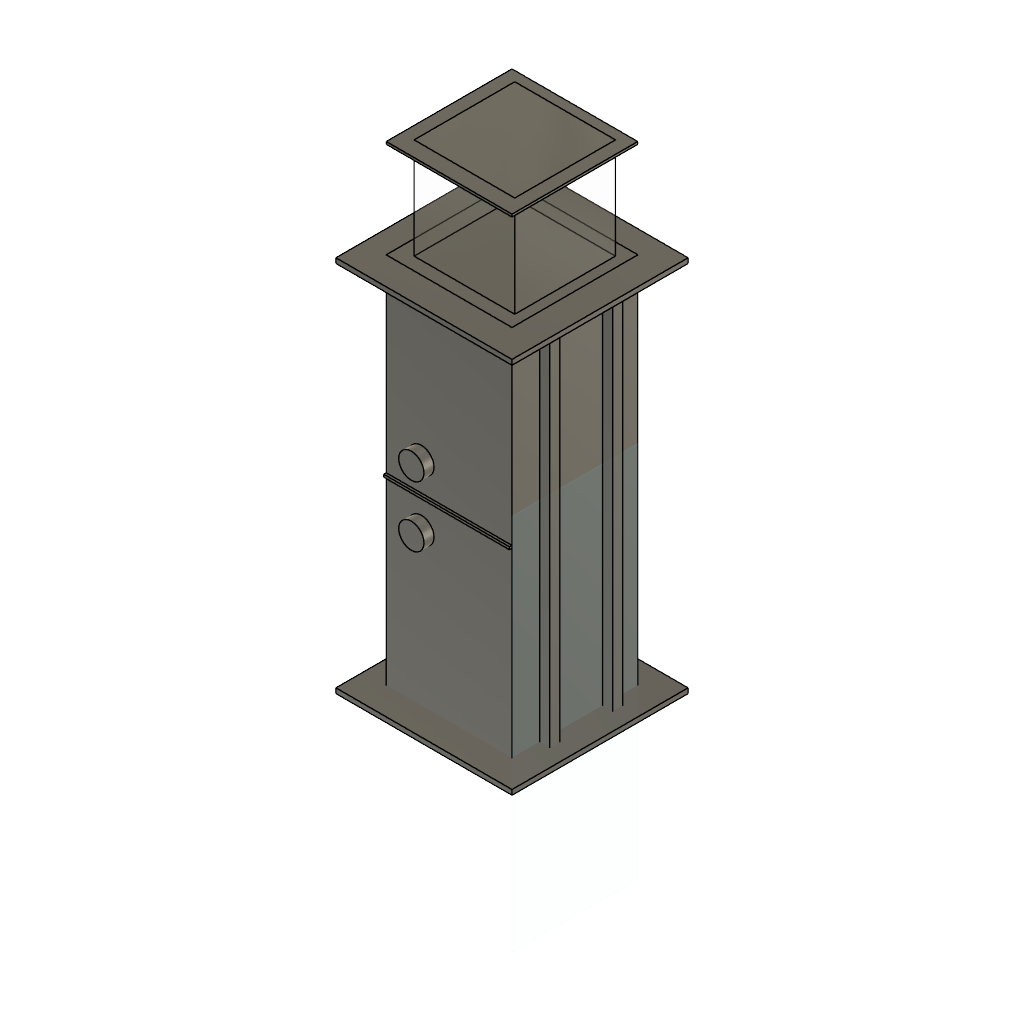
SolarPath+ (Autodesk Fusion 360 design; units mm, degrees)
Autodesk Fusion 360 part; units mm, degrees
sketch "Çizim1" plane through (0, 0, 0) normal (0, 1, 0) x (1, 0, 0)
  line L0 (0, 0) -> (250, 0)
  line L1 (250, 0) -> (250, 250)
  line L2 (250, 250) -> (0, 250)
  line L3 (0, 250) -> (0, 0)
  constraint horizontal L0
  constraint vertical L1
  constraint horizontal L2
  constraint vertical L3
  constraint coincident L0.start L3.end
extrude "Ekstrüzyon1" add sketch "Çizim1" along normal blind 750 makes body 1
move_body "Taşı1" bodies 1 to x (1, 0, 0) y (0, 1, 0) z (0, 0, 1) at (-125, 0, 250)
move_body "Taşı2" bodies 1 to x (1, 0, 0) y (0, 0, -1) z (0, 1, 0) at (0, 0, 0)
move_body "Taşı3" bodies 1 to x (1, 0, 0) y (0, 1, 0) z (0, 0, 1) at (0, -125, 750)
move_body "Taşı4" bodies 1 to x (1, 0, 0) y (0, 1, 0) z (0, 0, 1) at (0, 0, -325)
sketch "Çizim2" plane through (125, 0, 0) normal (1, 0, 0) x (0, 1, 0)
  line L0 (125, 425) -> (-125, 425)
  line L1 (-125, 425) -> (-125, -325)
  line L2 (-125, -325) -> (125, -325)
  line L3 (125, -325) -> (125, 425)
sketch "Çizim3" plane through (0, 0, 0) normal (0, 1, 0) x (1, 0, 0)
  line L0 (300, 150) -> (550, 150)
  line L1 (550, 150) -> (550, 155)
  line L2 (550, 155) -> (300, 155)
  line L3 (300, 155) -> (300, 150)
  constraint horizontal L0
  constraint vertical L1
  constraint horizontal L2
  constraint vertical L3
extrude "Ekstrüzyon2" add sketch "Çizim3" along normal blind 5 separate body makes body 2
sketch "Çizim4" plane through (0, 0, 0) normal (0, 1, 0) x (1, 0, 0)
move_body "Taşı5" bodies 2 to x (1, 0, 0) y (0, 1, 0) z (0, 0, 1) at (0, -135, 0)
move_body "Taşı6" bodies 2 to x (1, 0, 0) y (0, 1, 0) z (0, 0, 1) at (-425, 0, 0)
move_body "Taşı7" bodies 2 to x (1, 0, 0) y (0, 1, 0) z (0, 0, 1) at (0, 0, 150)
sketch "Çizim5" plane through (0, -125, 0) normal (0, -1, 0) x (1, 0, 0)
  line L0 (125, 425) -> (-125, 425)
  line L1 (-125, 425) -> (-125, -325)
  line L2 (-125, -325) -> (125, -325)
  line L3 (125, -325) -> (125, 425)
  line L4 (350, 0) -> (450, 0)
  line L5 (450, 0) -> (450, -35)
  line L6 (450, -35) -> (350, -35)
  line L7 (350, -35) -> (350, 0)
  dimension "d6" = 100
  dimension "d7" = 35
  constraint horizontal L4
  constraint vertical L5
  constraint horizontal L6
  constraint vertical L7
  measures "d6" distance of L4.start L4.end
  measures "d7" distance of L4.start L6.end
move_body "Taşı13" bodies 2 to x (1, 0, 0) y (0, 1, 0) z (0, 0, 1) at (0, 5, 70)
sketch "Çizim6" plane through (0, 0, 0) normal (0, 0, 1) x (1, 0, 0)
  line L0 (500, 150) -> (850, 150)
  line L1 (850, 150) -> (850, -200)
  line L2 (850, -200) -> (500, -200)
  line L3 (500, -200) -> (500, 150)
  constraint horizontal L0
  constraint vertical L1
  constraint horizontal L2
  constraint vertical L3
extrude "Ekstrüzyon4" add sketch "Çizim6" along normal blind 10 separate body makes body 3
move_body "Taşı16" bodies 3 to x (1, 0, 0) y (0, 1, 0) z (0, 0, 1) at (-670, 20, -330)
copy_body "Gövdeleri Kopyala Yapıştır2" bodies 3 makes body 4
move_body "Taşı17" bodies 4 to x (1, 0, 0) y (0, 1, 0) z (0, 0, 1) at (0, 0, 750)
sketch "Çizim7" plane through (0, 0, 0) normal (0, 1, 0) x (1, 0, 0)
  line L0 (450, 0) -> (650, 0)
  line L1 (650, 0) -> (650, -200)
  line L2 (650, -200) -> (450, -200)
  line L3 (450, -200) -> (450, 0)
  constraint horizontal L0
  constraint vertical L1
  constraint horizontal L2
  constraint vertical L3
extrude "Ekstrüzyon5" add sketch "Çizim7" along normal blind 200 separate body makes body 5
move_body "Taşı18" bodies 5 to x (1, 0, 0) y (0, 1, 0) z (0, 0, 1) at (-545, -99.5, 430)
sketch "Çizim8" plane through (0, 0, 0) normal (0, 1, 0) x (1, 0, 0)
  line L0 (500, 0) -> (750, 0)
  line L1 (750, 0) -> (750, -250)
  line L2 (750, -250) -> (500, -250)
  line L3 (500, -250) -> (500, 0)
  constraint horizontal L0
  constraint vertical L1
  constraint horizontal L2
  constraint vertical L3
extrude "Ekstrüzyon6" add sketch "Çizim8" along normal blind 5 separate body makes body 6
move_body "Taşı19" bodies 6 to x (1, 0, 0) y (0, 0, -1) z (0, 1, 0) at (0, -120, 130)
move_body "Taşı20" bodies 6 to x (1, 0, 0) y (0, 1, 0) z (0, 0, 1) at (-620, -10, 500)
move_body "Taşı21" bodies 3 to x (1, 0, 0) y (0, 1, 0) z (0, 0, 1) at (0, 0, 5)
move_body "Taşı22" bodies 4 to x (1, 0, 0) y (0, 1, 0) z (0, 0, 1) at (0, 0, -5)
move_body "Taşı23" bodies 5 to x (1, 0, 0) y (0, 1, 0) z (0, 0, 1) at (0, 0, -5)
move_body "Taşı24" bodies 6 to x (1, 0, 0) y (0, 1, 0) z (0, 0, 1) at (0, 0, -5)
sketch "Çizim9" plane through (0, 0, 0) normal (1, 0, 0) x (0, 1, 0)
sketch "Çizim10" plane through (0, 0, 0) normal (1, 0, 0) x (0, 1, 0)
  line L0 (500, 250) -> (520, 250)
  line L1 (520, 250) -> (520, -500)
  line L2 (520, -500) -> (500, -500)
  line L3 (500, -500) -> (500, 250)
  dimension "d16" = 20
  dimension "d17" = 750
  constraint horizontal L0
  constraint vertical L1
  constraint horizontal L2
  constraint vertical L3
  measures "d16" distance of L0.start L0.end
  measures "d17" distance of L0.start L2.end
sketch "Çizim11" plane through (0, 0, 0) normal (1, 0, 0) x (0, 1, 0)
  line L0 (-200, 420) -> (-220, 420)
  line L1 (-220, 420) -> (-220, -320)
  line L2 (-220, -320) -> (-200, -320)
  line L3 (-200, -320) -> (-200, 420)
  constraint horizontal L0
  constraint vertical L1
  constraint horizontal L2
  constraint vertical L3
extrude "Ekstrüzyon8" add sketch "Çizim11" along normal blind 20 separate body makes body 7
copy_body "Gövdeleri Kopyala Yapıştır7" bodies 7 makes body 8
move_body "Taşı32" bodies 8 to x (1, 0, 0) y (0, 1, 0) z (0, 0, 1) at (-200, 95, 0)
move_body "Taşı33" bodies 8 to x (1, 0, 0) y (0, 1, 0) z (0, 0, 1) at (0, 50, 0)
move_body "Taşı34" bodies 8 to x (1, 0, 0) y (0, 1, 0) z (0, 0, 1) at (55, 0, 0)
move_body "Taşı35" bodies 8 to x (1, 0, 0) y (0, 1, 0) z (0, 0, 1) at (5, 0, 0)
copy_body "Gövdeleri Kopyala Yapıştır8" bodies 7 makes body 9
move_body "Taşı36" bodies 9 to x (1, 0, 0) y (0, 1, 0) z (0, 0, 1) at (-145, 325, 0)
move_body "Taşı37" bodies 9 to x (1, 0, 0) y (0, 1, 0) z (0, 0, 1) at (0, -50, 0)
copy_body "Gövdeleri Kopyala Yapıştır9" bodies 7 makes body 10
move_body "Taşı38" bodies 10 to x (1, 0, 0) y (0, 1, 0) z (0, 0, 1) at (125, 100, 0)
move_body "Taşı39" bodies 10 to x (1, 0, 0) y (0, 1, 0) z (0, 0, 1) at (0, 50, 0)
copy_body "Gövdeleri Kopyala Yapıştır10" bodies 7 makes body 11
move_body "Taşı40" bodies 11 to x (1, 0, 0) y (0, 1, 0) z (0, 0, 1) at (200, 450, 0)
move_body "Taşı41" bodies 11 to x (1, 0, 0) y (0, 1, 0) z (0, 0, 1) at (-75, -125, 0)
move_body "Taşı42" bodies 11 to x (1, 0, 0) y (0, 1, 0) z (0, 0, 1) at (0, -50, 0)
move_body "Taşı43" bodies 7 to x (1, 0, 0) y (0, 1, 0) z (0, 0, 1) at (105, 345, 0)
move_body "Taşı44" bodies 7 to x (1, 0, 0) y (0, 1, 0) z (0, 0, 1) at (-50, 0, 0)
copy_body "Gövdeleri Kopyala Yapıştır11" bodies 7 makes body 12
move_body "Taşı45" bodies 12 to x (1, 0, 0) y (0, 1, 0) z (0, 0, 1) at (-180, 0, 0)
move_body "Taşı46" bodies 12 to x (1, 0, 0) y (0, 1, 0) z (0, 0, 1) at (50, 0, 0)
move_body "Taşı47" bodies 2 to x (1, 0, 0) y (0, 1, 0) z (0, 0, 1) at (0, 0, 3.55)
move_body "Taşı48" bodies 2 to x (1, 0, 0) y (0, 1, 0) z (0, 0, 1) at (0, -57, 351.45)
move_body "Taşı49" bodies 2 to x (1, 0, 0) y (0, 1, 0) z (0, 0, 1) at (0, 0, -375)
move_body "Taşı50" bodies 2 to x (1, 0, 0) y (0, 1, 0) z (0, 0, 1) at (0, 57, 0)
copy_body "Gövdeleri Kopyala Yapıştır13" bodies 2 makes body 13
sketch "Çizim12" plane through (0, 0, 0) normal (0, 1, 0) x (1, 0, 0)
  line L0 (150.0729, -50, 135) -> (190, -50, 135)
  line L1 (190, -50, 135) -> (190, -45, 135)
  line L2 (190, -45, 135) -> (150.0729, -45, 135)
  line L3 (150.0729, -45, 135) -> (150.0729, -50, 135)
sketch "Çizim13" plane through (0, -125, 0) normal (0, -1, 0) x (1, 0, 0)
  line L0 (125, 425) -> (-125, 425)
  line L1 (-125, 425) -> (-125, -325)
  line L2 (-125, -325) -> (125, -325)
  line L3 (125, -325) -> (125, 425)
  line L4 (415, 50) -> (433, 50)
  line L5 (433, 50) -> (433, 45)
  line L6 (433, 45) -> (415, 45)
  line L7 (415, 45) -> (415, 50)
  constraint horizontal L4
  constraint vertical L5
  constraint horizontal L6
  constraint vertical L7
sketch "Çizim14" plane through (0, 0, 0) normal (0, 1, 0) x (1, 0, 0)
sketch "Çizim15" plane through (0, 0, 0) normal (0, 1, 0) x (1, 0, 0)
  line L0 (413, -50, -232) -> (444, -50, -232)
  line L1 (444, -50, -232) -> (444, -45, -232)
  line L2 (444, -45, -232) -> (413, -45, -232)
  line L3 (413, -45, -232) -> (413, -50, -232)
sketch "Çizim16" plane through (0, -70, 0) normal (0, -1, 0) x (1, 0, 0)
  line L0 (125, 420) -> (125, -320)
  line L1 (125, -320) -> (145, -320)
  line L2 (145, -320) -> (145, 420)
  line L3 (145, 420) -> (125, 420)
  circle A0 centre (-500, 0) radius 25
extrude "Ekstrüzyon12" add sketch "Çizim16" along normal blind 20 separate body contours A0 makes body 14
move_face "YüzeyiTaşı2" to x (1, 0, 0) y (0, 1, 0) z (0, 0, 1) at (0, -90, 0) 1 faces at (-524.9689, -76.6667, 1.2461) on bodies 14
move_body "Taşı53" bodies 14 to x (1, 0, 0) y (0, 1, 0) z (0, 0, 1) at (0, -110, 0)
move_body "Taşı54" bodies 14 to x (1, 0, 0) y (0, 1, 0) z (0, 0, 1) at (0, 0, 47.1094)
move_body "Taşı55" bodies 14 to x (1, 0, 0) y (0, 1, 0) z (0, 0, 1) at (130, 55, 0)
move_body "Taşı57" bodies 14 to x (1, 0, 0) y (0, 1, 0) z (0, 0, 1) at (290, 0, 60)
copy_body "Gövdeleri Kopyala Yapıştır15" bodies 14 makes body 15
copy_body "Gövdeleri Kopyala Yapıştır16" bodies 14 makes body 16
move_body "Taşı58" bodies 16 to x (1, 0, 0) y (0, 1, 0) z (0, 0, 1) at (0, 0, -140.44)
move_body "Taşı59" bodies 16 to x (1, 0, 0) y (0, 1, 0) z (0, 0, 1) at (0, 0, 20)
move_body "Taşı60" bodies 14 15 to x (1, 0, 0) y (0, 1, 0) z (0, 0, 1) at (25, 0, 0)
move_body "Taşı61" bodies 16 to x (1, 0, 0) y (0, 1, 0) z (0, 0, 1) at (25, 0, 0)
move_body "Taşı62" bodies 11 10 5 4 16 1 3 14 9 6 13 12 15 2 8 7 to x (1, 0, 0) y (0, 1, 0) z (0, 0, 1) at (0, 0, 325)
